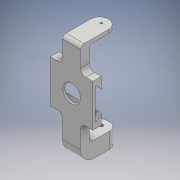
# Autodesk Inventor part: InnerFrame
Saved by Autodesk Inventor 2017 (Build 210142000, 142)
## iProperties
Created: 2016-05-22
Part Number: InnerFrame
Material: Generic
Document SubType Name: Modeling
Designer: Kurtis
Density: 1 g/cm^3
Appearance: Default
Author: Kurtis
Autodesk Inventor part; units mm, degrees
ref_plane "YZ Plane" through (0, 0, 0) normal (1, 0, 0) x (0, 1, 0)
ref_plane "XZ Plane" through (0, 0, 0) normal (0, 1, 0) x (-1, 0, 0)
ref_plane "XY Plane" through (0, 0, 0) normal (0, 0, 1) x (1, 0, 0)
sketch "Sketch1" plane through (0, 0, 0) normal (0, 0, 1) x (1, 0, 0)
  line L0 (-30, -6) -> (30, -6)
  line L1 (30, -6) -> (30, 6)
  line L2 (30, 6) -> (-30, 6)
  line L3 (-30, 6) -> (-30, -6)
  line L4 (-30, -6) -> (30, 6) construction
  line L5 (30, -6) -> (-30, 6) construction
  line L6 (30, 6) -> (25, 6) construction
  line L7 (-30, 6) -> (-25, 6) construction
  point P0 (0, 0)
  dimension "d0" = 60
  dimension "d1" = 12
  constraints: 16 end point, 2 midpoint, 2 parallel, 2 point on line, 1 horizontal, 1 perpendicular
  measures "d0" distance of L2.end L1.end
  measures "d1" distance of L1.end L0.end
extrude "Block" add sketch "Sketch1" along normal blind 60
sketch "Sketch2" plane through (30, -6, 0) normal (1, 0, 0) x (0, 0, -1)
  line L0 (0, 12) -> (-60, 12) projected
  line L1 (-30, 12) -> (-15.25, 12)
  line L2 (-30, 12) -> (-44.75, 12)
  line L3 (-30, 12) -> (-30, 3.1) construction
  line L4 (-30, 3.1) -> (-8.25, 3.1)
  line L5 (-30, 3.1) -> (-51.75, 3.1)
  line L6 (-51.75, 3.1) -> (-51.75, 5.1)
  line L7 (-8.25, 3.1) -> (-8.25, 5.1)
  line L8 (-8.25, 5.1) -> (-15.25, 12)
  line L9 (-51.75, 5.1) -> (-44.75, 12)
  point P0 (0, 6)
  dimension "d17" = 14.75
  dimension "d18" = 14.75
  dimension "d19" = 8.9
  dimension "d20" = 21.75
  dimension "d21" = 21.75
  dimension "d22" = 2
  dimension "d23" = 2
  constraints: 18 end point, 2 perpendicular, 2 point on line, 2 vertical, 1 horizontal, 1 midpoint
  measures "d17" distance of L1.start L1.end
  measures "d18" distance of L1.start L2.end
  measures "d19" distance of L1.start L3.end
  measures "d20" distance of L3.end L4.end
  measures "d21" distance of L3.end L5.end
  measures "d22" distance of L5.end L6.end
  measures "d23" distance of L4.end L7.end
extrude "Tripod Slot" cut sketch "Sketch2" against normal blind 60
hole "Hole1" at (0, -2.9, 30) direction (0, -1, 0) diameter 22.5 end through all
sketch "Sketch4" plane through (0, 0, 0) normal (0, 0, -1) x (-1, 0, 0)
  line L0 (-30, 6) -> (30, 6) projected
  line L1 (-12.7, -6) -> (12.7, -6)
  line L2 (12.7, -6) -> (12.7, 6)
  line L3 (12.7, 6) -> (-12.7, 6)
  line L4 (-12.7, 6) -> (-12.7, -6)
  line L5 (-12.7, -6) -> (12.7, 6) construction
  line L6 (12.7, -6) -> (-12.7, 6) construction
  point P0 (0, 0)
  dimension "d64" = 25.4
  dimension "d65" = 25.288
  dimension "d66" = 17.3
  constraints: 12 end point, 2 midpoint, 2 parallel, 1 horizontal, 1 perpendicular, 1 point on line
  measures "d64" distance of L3.end L2.end
  measures "d65" angle of L5 L0
  measures "d66" distance from line of L0.end L2
extrude "Extrusion4" add sketch "Sketch4" along normal blind 52.5
sketch "Sketch5" plane through (-30, 6, 15.25) normal (0, 1, 0) x (1, 0, 0)
  line L0 (60, -29.5) -> (60, 0) projected
  line L1 (17.3, 67.75) -> (42.7, 67.75) projected
  line L2 (42.7, 15.25) -> (42.7, 67.75) projected
  line L3 (17.3, 67.75) -> (42.7, 67.75)
  line L4 (42.7, 67.75) -> (42.7, 45.25)
  line L5 (42.7, 45.25) -> (17.3, 45.25)
  line L6 (17.3, 45.25) -> (17.3, 67.75)
  line L7 (17.3, 15.25) -> (17.3, 67.75) construction
  line L8 (42.7, 45.25) -> (17.3, 67.75) construction
  circle A0 centre (30, 56.5) radius 1.5
  point P0 (30, 15.25)
  dimension "d67" = 22.5
  dimension "d68" = 3
  constraints: 10 end point, 2 parallel, 1 centre point, 1 horizontal, 1 midpoint, 1 perpendicular, 1 point on line
  measures "d67" distance of L3.end L4.end
  measures "d68" diameter of A0
extrude "Extrusion5" add sketch "Sketch5" along normal blind 40
sketch "Sketch6" plane through (0, 0, -52.5) normal (0, 0, -1) x (-1, 0, 0)
  line L0 (0, 0) -> (0, 46) construction
  circle A0 centre (0, 36) radius 2.5
  line L1 (-12.7, 46) -> (12.7, 46) construction
  line L2 (-12.7, 46) -> (12.7, 46) construction
  line L3 (12.7, 46) -> (0, 46) construction
  line L4 (0, 36) -> (0, 46) construction
  dimension "d60" = 5
  dimension "d61" = 10
  constraints: 8 end point, 3 collinear, 1 centre point, 1 point on line
  measures "d60" diameter of A0
  measures "d61" distance of L0.end L4.start
extrude "Extrusion6" cut sketch "Sketch6" against normal blind 31.75
fillet "Fillet4" radius 11 2 edges at (12.7, 46, -41.25) (-12.7, 46, -41.25)
fillet "Fillet5" radius 20 1 edges at (0, -6, -52.5)
fillet "Fillet6" radius 5 1 edges at (0, 6, -30)
sketch "Sketch7" plane through (0, 0, 60) normal (0, 0, 1) x (1, 0, 0)
  line L0 (-30, 6) -> (30, 6) projected
  line L1 (-12.7, -6) -> (12.7, -6)
  line L2 (12.7, -6) -> (12.7, 6)
  line L3 (12.7, 6) -> (-12.7, 6)
  line L4 (-12.7, 6) -> (-12.7, -6)
  line L5 (-12.7, -6) -> (12.7, 6) construction
  line L6 (12.7, -6) -> (-12.7, 6) construction
  point P0 (0, 0)
  dimension "d73" = 25.4
  constraints: 12 end point, 2 midpoint, 2 parallel, 1 horizontal, 1 perpendicular, 1 point on line
  measures "d73" distance of L3.end L2.end
extrude "Extrusion7" add sketch "Sketch7" along normal blind 35
sketch "Sketch8" plane through (-30, 6, 44.75) normal (0, 1, 0) x (1, 0, 0)
  line L0 (30, -50.25) -> (30, 0) construction
  line L1 (60, 0) -> (0, 0) construction
  line L2 (30, -50.25) -> (30, -47.75) construction
  line L3 (17.3, -15.25) -> (17.3, -50.25) projected
  line L4 (42.7, -50.25) -> (17.3, -50.25)
  line L5 (17.3, -50.25) -> (17.3, -45.25)
  line L6 (17.3, -45.25) -> (42.7, -45.25)
  line L7 (42.7, -45.25) -> (42.7, -50.25)
  line L8 (42.7, -50.25) -> (17.3, -45.25) construction
  line L9 (17.3, -50.25) -> (42.7, -45.25) construction
  point P0 (30, 44.75)
  dimension "d76" = 2.5
  dimension "d81" = 5
  constraints: 16 end point, 3 midpoint, 2 parallel, 2 point on line, 1 horizontal, 1 perpendicular
  measures "d76" distance of L0.start L2.end
  measures "d81" distance of L4.end L5.end
extrude "Extrusion8" add sketch "Sketch8" along normal blind 40
hole "Hole2" at (0, 36, 95) direction (0, 0, -1) diameter 3 end through all
fillet "Fillet7" radius 12.7 2 edges at (12.7, 46, 92.5) (-12.7, 46, 92.5)
fillet "Fillet8" radius 5 1 edges at (0, 6, 90)
fillet "Fillet9" radius 5 1 edges at (0, -6, 95)
fillet "Fillet10" radius 7.5 4 edges at (12.7, 0, 0) (-12.7, 0, 0) (-12.7, 0, 60) (12.7, 0, 60)
fillet "Fillet11" radius 1.5 2 edges at (0, -6, 18.75) (0, -2.9, 18.75)
body "Solid1"
